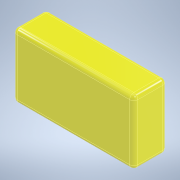
# Autodesk Inventor part: Bateria 3S 650mAh
Saved by Autodesk Inventor 2021 (Build 250183000, 183)
## iProperties
Created: 2022-10-29
Part Number: Bateria 3S 650mAh
Material: Genérico
Document SubType Name: Modeling
Designer: nicho
Mass: 59 g
Surface Area: 60.7894 cm^2
Volume: 28.4182 cm^3
Density: 2.07614 g/cm^3
Appearance: Amarelo
Author: nicho
Autodesk Inventor part; units mm, degrees
ref_plane "YZ Plane" through (0, 0, 0) normal (1, 0, 0) x (0, 1, 0)
ref_plane "XZ Plane" through (0, 0, 0) normal (0, 1, 0) x (-1, 0, 0)
ref_plane "XY Plane" through (0, 0, 0) normal (0, 0, 1) x (1, 0, 0)
sketch "Esboço1" plane through (0, 0, 0) normal (0, 1, 0) x (-1, 0, 0)
  line L0 (-29, 8) -> (29, 8)
  line L1 (29, 8) -> (29, -8)
  line L2 (29, -8) -> (-29, -8)
  line L3 (-29, -8) -> (-29, 8)
  line L4 (-29, 8) -> (29, -8) construction
  line L5 (29, 8) -> (-29, -8) construction
  point P0 (0, 0)
  dimension "d0" = 58
  dimension "d1" = 16
  constraints: 12 end point, 2 midpoint, 2 parallel, 1 horizontal, 1 perpendicular
  measures "d0" distance of L1.end L2.end
  measures "d1" distance of L0.end L1.end
extrude "Extrusão1" add sketch "Esboço1" along normal blind 31
fillet "Arredondamento1" radius 2 12 edges at (29, 15.5, 8) (29, 31, 0) (0, 31, 8) (29, 15.5, -8) (0, 31, -8) (29, 0, 0) (0, 0, 8) (0, 0, -8) (-29, 0, 0) (-29, 15.5, -8) (-29, 15.5, 8) (-29, 31, 0)
